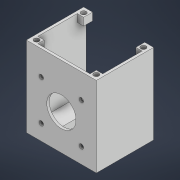
# Autodesk Inventor part: Motorhalterung_v2
Saved by Autodesk Inventor 2021 (Build 250183000, 183)
## iProperties
Created: 2021-01-03
Part Number: Motorhalterung_v2
Material: Generisch
Document SubType Name: Modeling
Designer: Ctroi
Density: 1 g/cm^3
Appearance: Vorgabe
Mass: 18.8981 g
Surface Area: 175.763 cm^2
Volume: 18.8981 cm^3
Author: Ctroi
## iProperties of the stored document _3D-Druck.ipt
Created: 2021-01-07
Part Number: _3D-Druck
Material: Generisch
Document SubType Name: Modeling
Designer: Ctroi
Density: 1 g/cm^3
Appearance: Vorgabe
Author: Ctroi
Autodesk Inventor part; units mm, degrees
ref_plane "YZ Plane" through (0, 0, 0) normal (1, 0, 0) x (0, 1, 0)
ref_plane "XZ Plane" through (0, 0, 0) normal (0, 1, 0) x (-1, 0, 0)
ref_plane "XY Plane" through (0, 0, 0) normal (0, 0, 1) x (1, 0, 0)
sketch "Skizze1" plane through (0, 0, 0) normal (0, 1, 0) x (-1, 0, 0)
  line L0 (-27.5, 22.5) -> (27.5, 22.5)
  line L1 (27.5, 22.5) -> (27.5, -22.5)
  line L2 (27.5, -22.5) -> (-27.5, -22.5)
  line L3 (-27.5, -22.5) -> (-27.5, 22.5)
  line L4 (0, -31.5) -> (0, 31.5) projected
  line L5 (38.5, 0) -> (-38.5, 0) projected
  point P0 (0, 0)
  dimension "d0" = 55
  dimension "d1" = 45
  constraints: 8 end point, 2 parallel, 1 horizontal, 1 perpendicular, 2 other
  measures "d0" distance of L1.end L2.end
  measures "d1" distance of L0.end L1.end
extrude "Extrusion1" add sketch "Skizze1" along normal blind 3
sketch "Skizze2" plane through (0, 3, 0) normal (0, 1, 0) x (1, 0, 0)
  line L0 (-27.5, 22.5) -> (-27.5, -22.5) projected
  line L1 (27.5, -22.5) -> (27.5, 22.5) projected
  line L2 (-27.5, -22.5) -> (27.5, -22.5)
  line L3 (27.5, -22.5) -> (27.5, -20.5)
  line L4 (27.5, -20.5) -> (-27.5, -20.5)
  line L5 (-27.5, -20.5) -> (-27.5, -22.5)
  point P0 (0, 0)
  dimension "d4" = 2
  constraints: 8 end point, 2 parallel, 1 horizontal, 1 perpendicular, 1 point on line
  measures "d4" distance of L3.end L2.end
extrude "Extrusion2" add sketch "Skizze2" along normal blind 57
sketch "Skizze3" plane through (-27.5, 0, 22.5) normal (0, 0, 1) x (1, 0, 0)
  circle A0 centre (27.5, 25) radius 11.5
  line L0 (0, 0) -> (55, 0) projected
  line L1 (55, 0) -> (55, 60) projected
  circle A1 centre (43.25, 9.25) radius 1.75
  circle A2 centre (11.75, 9.25) radius 1.75
  circle A3 centre (11.75, 40.75) radius 1.75
  circle A4 centre (43.25, 40.75) radius 1.75
  line L2 (0, 60) -> (55, 60) projected
  line L3 (27.5, 60) -> (27.5, 0)
  line L4 (4.6208, 25) -> (55, 25)
  dimension "d7" = 23
  dimension "d10" = 3.5
  dimension "d11" = 3.5
  dimension "d12" = 3.5
  dimension "d13" = 3.5
  dimension "d17" = 31.5
  dimension "d48" = 0
  constraints: 5 centre point, 4 end point, 3 symmetric about line, 2 perpendicular, 1 midpoint, 1 point on line
  measures "d7" diameter of A0
  measures "d10" diameter of A1
  measures "d11" diameter of A2
  measures "d12" diameter of A3
  measures "d13" diameter of A4
  measures "d17" diameter of A4.centre L3
  measures "d48" distance from line of A0.centre L3
extrude "Extrusion3" cut sketch "Skizze3" against normal up to surface (2 mm away) contours L4 L3 A0 | A0 L3 L4 | L3 L4 A0 | A0 L4 L3 | A1 | A2 | A3 | A4
sketch "Skizze10" plane through (0, 3, 0) normal (0, 1, 0) x (1, 0, 0)
  line L0 (27.5, -20.5) -> (27.5, 22.5) projected
  line L1 (27.5, 22.5) -> (-27.5, 22.5) projected
  line L2 (27.5, -20.5) -> (25.5, -20.5)
  line L3 (25.5, -20.5) -> (25.5, 22.5)
  line L4 (25.5, 22.5) -> (27.5, 22.5)
  line L5 (27.5, 22.5) -> (27.5, -20.5)
  line L6 (27.5, -20.5) -> (-27.5, -20.5) projected
  line L7 (-27.5, 22.5) -> (-25.5, 22.5)
  line L8 (-25.5, 22.5) -> (-25.5, -20.5)
  line L9 (-25.5, -20.5) -> (-27.5, -20.5)
  line L10 (-27.5, -20.5) -> (-27.5, 22.5)
  point P0 (0, 0)
  point P1 (-27.5, -20.5)
  dimension "d43" = 2
  dimension "d44" = 2
  constraints: 16 end point, 4 parallel, 2 horizontal, 2 perpendicular, 2 point on line
  measures "d43" distance of L3.end L4.end
  measures "d44" distance of L8.end L9.end
extrude "Extrusion6" add sketch "Skizze10" along normal blind 57 contours L2 L3 L1 L0 | L6 L10 L1 L8
sketch "Skizze11" plane through (0, 0, 0) normal (0, -1, 0) x (1, 0, 0)
  line L0 (27.5, 22.5) -> (27.5, -22.5) projected
  line L1 (-27.5, 22.5) -> (27.5, 22.5) projected
  line L2 (27.5, -22.5) -> (-27.5, -22.5)
  line L3 (-27.5, -22.5) -> (-27.5, 22.5)
  line L4 (-27.5, 22.5) -> (27.5, 22.5)
  line L5 (27.5, 22.5) -> (27.5, -22.5)
  point P0 (0, 0)
  constraints: 8 end point, 2 parallel, 1 horizontal, 1 perpendicular
extrude "Extrusion7" add sketch "Skizze11" along normal blind 3
sketch "Skizze12" plane through (0, 3, 0) normal (0, 1, 0) x (1, 0, 0)
  circle A0 centre (15, -15) radius 2
  circle A1 centre (-15, -15) radius 2
  circle A2 centre (15, 15) radius 2
  circle A3 centre (-15, 15) radius 2
  line L0 (0, 31.5) -> (0, -31.5) projected
  line L1 (-38.5, 0) -> (38.5, 0) projected
  point P0 (0, 0)
  dimension "d52" = 4
  dimension "d53" = 4
  dimension "d54" = 4
  dimension "d55" = 4
  dimension "d56" = 30
  dimension "d57" = 30
  constraints: 4 centre point, 4 symmetric about line
  measures "d52" diameter of A0
  measures "d53" diameter of A1
  measures "d54" diameter of A2
  measures "d55" diameter of A3
  measures "d56" distance of A0.centre A2.centre
  measures "d57" distance of A3.centre A2.centre
extrude "Extrusion8" cut sketch "Skizze12" against normal up to surface (6 mm away)
sketch "Skizze13" plane through (0, 60, 0) normal (0, 1, 0) x (1, 0, 0)
  line L0 (25.5, -20.5) -> (20.5, -20.5)
  line L1 (20.5, -20.5) -> (20.5, -15.5)
  line L2 (20.5, -15.5) -> (25.5, -15.5)
  line L3 (25.5, -15.5) -> (25.5, -20.5)
  line L4 (-25.5, 22.5) -> (-25.5, -20.5) projected
  line L5 (-25.5, -20.5) -> (-20.5, -20.5)
  line L6 (-20.5, -20.5) -> (-20.5, -15.5)
  line L7 (-20.5, -15.5) -> (-25.5, -15.5)
  line L8 (-25.5, -15.5) -> (-25.5, -20.5)
  line L9 (25.5, 22.5) -> (20.5, 22.5)
  line L10 (20.5, 22.5) -> (20.5, 15.5)
  line L11 (20.5, 15.5) -> (25.5, 15.5)
  line L12 (25.5, 15.5) -> (25.5, 22.5)
  line L13 (25.5, 22.5) -> (-25.5, 22.5) projected
  line L14 (-25.5, 22.5) -> (-20.5, 22.5)
  line L15 (-20.5, 22.5) -> (-20.5, 15.5)
  line L16 (-20.5, 15.5) -> (-25.5, 15.5)
  line L17 (-25.5, 15.5) -> (-25.5, 22.5)
  point P0 (0, 0)
  point P1 (-25.5, -15.5)
  dimension "d60" = 5
  dimension "d61" = 5
  dimension "d62" = 5
  dimension "d63" = 5
  dimension "d64" = 5
  dimension "d65" = 7
  dimension "d66" = 5
  dimension "d67" = 7
  constraints: 32 end point, 8 parallel, 4 horizontal, 4 perpendicular, 1 point on line
  measures "d60" distance of L1.end L2.end
  measures "d61" distance of L0.end L1.end
  measures "d62" distance of L7.end L6.end
  measures "d63" distance of L6.end L5.end
  measures "d64" distance of L11.end L10.end
  measures "d65" distance of L10.end L9.end
  measures "d66" distance of L15.end L16.end
  measures "d67" distance of L14.end L15.end
sketch "Skizze15" plane through (0, -3, 0) normal (0, -1, 0) x (1, 0, 0)
  line L0 (-27.5, -22.5) -> (27.5, -22.5) projected
  line L1 (-25.5, 20.5) -> (25.5, 20.5) projected
  line L2 (11.5, -22.5) -> (-11.5, -22.5)
  line L3 (-11.5, -22.5) -> (-11.5, 20.5)
  line L4 (-11.5, 20.5) -> (11.5, 20.5)
  line L5 (11.5, 20.5) -> (11.5, -22.5)
  line L6 (0, 31.5) -> (0, -31.5) projected
  line L7 (-38.5, 0) -> (38.5, 0) projected
  circle A0 centre (15, -15) radius 2 projected
  point P0 (0, 0)
  point P1 (11.5, 20.5)
  dimension "d94" = 1.5
  constraints: 8 end point, 2 parallel, 2 point on line, 1 horizontal, 1 perpendicular, 1 other
  measures "d94" distance edge to line of A0 L5
extrude "Extrusion11" cut sketch "Skizze15" against normal up to surface (6 mm away) contours L3 L7 L6 L0 | L6 L7 L5 L0 | L3 L1 L6 L7 | L6 L1 L5 L7
extrude "Extrusion12" add sketch "Skizze13" against normal blind 6
sketch "Skizze16" plane through (0, 60, 0) normal (0, 1, 0) x (1, 0, 0)
  line L0 (38.5, 0) -> (-38.5, 0) projected
  line L1 (0, 31.5) -> (0, -31.5) projected
  circle A0 centre (23.5, -18.5) radius 2
  circle A1 centre (-23.5, -18.5) radius 2
  circle A2 centre (-23.5, 18.5) radius 2
  circle A3 centre (23.5, 18.5) radius 2
  line L2 (-27.5, -22.5) -> (27.5, -22.5) projected
  line L3 (27.5, -22.5) -> (27.5, 22.5) projected
  line L4 (27.5, 22.5) -> (20.5, 22.5) projected
  line L5 (-20.5, 22.5) -> (-27.5, 22.5) projected
  line L6 (-27.5, 22.5) -> (-27.5, -22.5) projected
  point P0 (0, 0)
  dimension "d100" = 4
  dimension "d101" = 4
  dimension "d102" = 4
  dimension "d103" = 4
  dimension "d104" = 4
  dimension "d105" = 4
  dimension "d106" = 4
  dimension "d107" = 4
  dimension "d108" = 4
  dimension "d109" = 4
  dimension "d110" = 4
  dimension "d111" = 4
  constraints: 4 centre point
  measures "d100" diameter of A0
  measures "d101" diameter of A1
  measures "d102" diameter of A2
  measures "d103" diameter of A3
  measures "d104" distance from line of L2 A0.centre
  measures "d105" distance from line of L3 A0.centre
  measures "d106" distance from line of L4 A3.centre
  measures "d107" distance from line of L3 A3.centre
  measures "d108" distance from line of L5 A2.centre
  measures "d109" distance from line of L6 A1.centre
  measures "d110" distance from line of L2 A1.centre
  measures "d111" distance from line of L6 A2.centre
extrude "Extrusion13" cut sketch "Skizze16" against normal up to surface (6 mm away) contours A0 | A1 | A2 | A3
